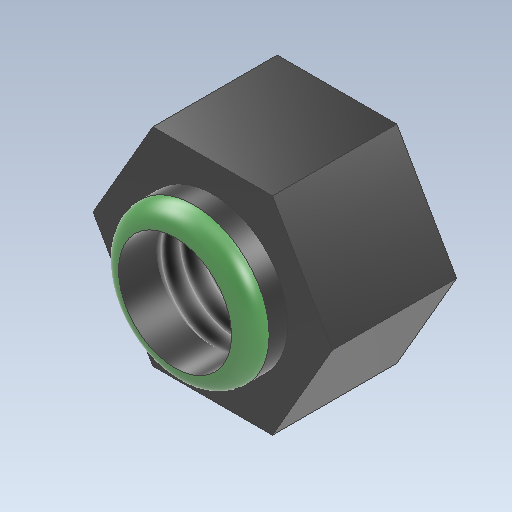
# Autodesk Inventor part: ナットナイロンM3
Saved by Autodesk Inventor 2020.2 (Build 242310000, 310)
## iProperties
Created: 2020-02-25
Part Number: ナットナイロンM3
Material: 鋼
Document SubType Name: Modeling
Designer: aoyam
Density: 7.85 g/cm^3
Appearance: サテン - 黒
Author: aoyam
Autodesk Inventor part; units mm, degrees
ref_plane "YZ Plane" through (0, 0, 0) normal (1, 0, 0) x (0, 1, 0)
ref_plane "XZ Plane" through (0, 0, 0) normal (0, 1, 0) x (-1, 0, 0)
ref_plane "XY Plane" through (0, 0, 0) normal (0, 0, 1) x (1, 0, 0)
sketch "スケッチ1" plane through (0, 0, 0) normal (0, 0, 1) x (1, 0, 0)
  line L0 (-1.5877, 2.75) -> (1.5877, 2.75)
  line L1 (1.5877, 2.75) -> (3.1754, 0)
  line L2 (3.1754, 0) -> (1.5877, -2.75)
  line L3 (1.5877, -2.75) -> (-1.5877, -2.75)
  line L4 (-1.5877, -2.75) -> (-3.1754, 0)
  line L5 (-3.1754, 0) -> (-1.5877, 2.75)
  circle A0 centre (0, 0) radius 1.5
  point P0 (0, 0)
  point P1 (0, 0)
  dimension "d0" = 5.5
  dimension "d1" = 3
  constraints: 12 end point, 1 centre point, 1 coincident, 1 horizontal, 13 other
  measures "d0" distance between parallel lines of L3 L0
  measures "d1" diameter of A0
extrude "押し出し1" add sketch "スケッチ1" along normal blind 3.3
sketch "スケッチ2" plane through (0, 0, 3.3) normal (0, 0, 1) x (1, 0, 0)
  circle A0 centre (0, 0) radius 1.5 projected
  circle A1 centre (0, 0) radius 2
  point P0 (0, 0)
  dimension "d4" = 0.5
  constraints: 1 centre point
  measures "d4" radial gap between concentric circles of A0 A1
extrude "押し出し2" add sketch "スケッチ2" along normal blind 1
thread "ねじ1" size "M3x0.5" class "6H" standard "ANSI Metric M Profile" length 3.3
fillet "フィレット1" radius 0.5 1 edges at (-2, 0, 4.3)
